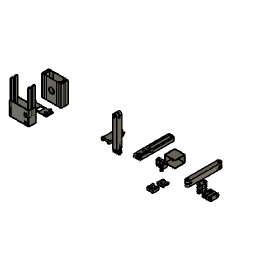
Table Lamp 3.0 v83 (Autodesk Fusion 360 design; units mm, degrees)
Autodesk Fusion 360 part; units mm, degrees
(part 1 of 3)
sketch "Schizzo1" plane through (0, 0, 0) normal (0, 0, 1) x (1, 0, 0)
  line L0 (-21, 0) -> (-5, 0)
  line L1 (-5, 0) -> (-5, 140)
  line L2 (-5, 140) -> (-21, 140)
  line L3 (-21, 140) -> (-21, 0)
  line L4 (-13, 140) -> (-13, 0)
  circle A0 centre (-13, 8) radius 8
  circle A1 centre (-13, 8) radius 4.1
  line L5 (-21, 70) -> (-5, 70)
  circle A2 centre (-13, 132) radius 8
  circle A3 centre (-13, 132) radius 4.1
  line L6 (26.1674, 0.6558) -> (42.1674, 0.6558)
  line L7 (42.1674, 0.6558) -> (42.1674, 33.6558)
  line L8 (42.1674, 33.6558) -> (26.1674, 33.6558)
  line L9 (26.1674, 33.6558) -> (26.1674, 0.6558)
  line L10 (34.1674, 0.6558) -> (34.1674, 33.6558)
  line L11 (26.1674, 17.1558) -> (42.1674, 17.1558)
  circle A4 centre (34.1674, 8.6558) radius 8
  arc A5 (42.1674, 11.5281) -> (34.1674, 17.1558) centre (34.1674, 8.6558) ccw
  circle A6 centre (34.1674, 25.6558) radius 8
  arc A7 (34.1674, 17.1558) -> (42.1674, 22.7835) centre (34.1674, 25.6558) ccw
  circle A8 centre (34.1674, 8.6558) radius 3.25
  line L12 (37.4174, 8.6519) -> (35.7958, 11.4684)
  line L13 (35.7958, 11.4684) -> (32.5458, 11.4724)
  line L14 (32.5458, 11.4724) -> (30.9174, 8.6597)
  line L15 (30.9174, 8.6597) -> (32.539, 5.8432)
  line L16 (32.539, 5.8432) -> (35.789, 5.8393)
  line L17 (35.789, 5.8393) -> (37.4174, 8.6519)
  line L18 (30.9174, 25.6519) -> (32.539, 28.4684)
  line L19 (32.539, 28.4684) -> (35.789, 28.4724)
  line L20 (35.789, 28.4724) -> (37.4174, 25.6597)
  line L21 (37.4174, 25.6597) -> (35.7958, 22.8432)
  line L22 (35.7958, 22.8432) -> (32.5458, 22.8393)
  line L23 (32.5458, 22.8393) -> (30.9174, 25.6519)
  circle A9 centre (34.1674, 8.6558) radius 1.6
  circle A10 centre (34.1674, 25.6558) radius 1.6
  circle A11 centre (-13, 8) radius 2
  circle A12 centre (-13, 132) radius 2
  line L24 (-130.5, 0) -> (-102.5, 0)
  line L25 (-102.5, 0) -> (-102.5, 16)
  line L26 (-102.5, 16) -> (-130.5, 16)
  line L27 (-130.5, 16) -> (-130.5, 0)
  line L28 (-116.5, 16) -> (-116.5, 0)
  line L29 (-130.5, 8) -> (-102.5, 8)
  line L30 (-130.5, 16) -> (-126.5, 16)
  line L31 (-126.5, 16) -> (-126.5, 0)
  line L32 (-126.5, 0) -> (-130.5, 0)
  line L33 (-130.5, 0) -> (-130.5, 16)
  line L34 (-106.5, 16) -> (-106.5, 0)
  line L35 (-115, 0) -> (-118, 0)
  line L36 (-118, 0) -> (-118, 16)
  line L37 (-118, 16) -> (-115, 16)
  line L38 (-115, 16) -> (-115, 0)
  line L39 (-115, 0) -> (-118, 16) construction
  line L40 (-118, 0) -> (-115, 16) construction
  line L41 (-114.5, 6) -> (-118.5, 6)
  line L42 (-118.5, 6) -> (-118.5, 10)
  line L43 (-118.5, 10) -> (-114.5, 10)
  line L44 (-114.5, 10) -> (-114.5, 6)
  line L45 (-114.5, 6) -> (-118.5, 10) construction
  line L46 (-118.5, 6) -> (-114.5, 10) construction
  line L47 (-114.5, 6) -> (-118.5, 6)
  line L48 (-118.5, 6) -> (-118.5, 10)
  line L49 (-118.5, 10) -> (-114.5, 10)
  line L50 (-114.5, 10) -> (-114.5, 6)
  line L51 (-114.5, 6) -> (-118.5, 10) construction
  line L52 (-118.5, 6) -> (-114.5, 10) construction
  circle A13 centre (-116.5, 8) radius 2.5
  line L53 (-135.9612, 39.7916) -> (-95.9612, 39.7916)
  line L54 (-95.9612, 39.7916) -> (-95.9612, 79.7916)
  line L55 (-95.9612, 79.7916) -> (-135.9612, 79.7916)
  line L56 (-135.9612, 79.7916) -> (-135.9612, 39.7916)
  circle A14 centre (-116.5, 8) radius 5
  circle A15 centre (-127.9112, 65.7416) radius 5.05
  line L57 (-132.9612, 79.7916) -> (-132.9612, 39.7916) construction
  line L58 (-135.9612, 79.7916) -> (-133.9612, 79.7916)
  line L59 (-133.9612, 79.7916) -> (-133.9612, 39.7916)
  line L60 (-133.9612, 39.7916) -> (-135.9612, 39.7916)
  line L61 (-135.9612, 39.7916) -> (-135.9612, 79.7916)
  line L62 (-135.9612, 79.7916) -> (-95.9612, 79.7916)
  line L63 (-95.9612, 79.7916) -> (-95.9612, 77.7916)
  line L64 (-95.9612, 77.7916) -> (-135.9612, 77.7916)
  line L65 (-135.9612, 77.7916) -> (-135.9612, 79.7916)
  line L66 (-135.9612, 70.7916) -> (-95.9612, 70.7916) construction
  line L67 (-95.9612, 65.7416) -> (-135.9612, 65.7416) construction
  line L68 (-78.8911, -24.4102) -> (-54.8911, -24.4102)
  line L69 (-54.8911, -24.4102) -> (-54.8911, -48.4102)
  line L70 (-54.8911, -48.4102) -> (-78.8911, -48.4102)
  line L71 (-78.8911, -48.4102) -> (-78.8911, -24.4102)
  line L72 (-78.8911, -38.4102) -> (-54.8911, -38.4102) construction
  line L73 (-75.8911, -24.4102) -> (-75.8911, -48.4102) construction
  circle A16 centre (-75.8911, -38.4102) radius 1.6
  line L74 (-66.8911, -24.4102) -> (-66.8911, -48.4102) construction
  circle A17 centre (-57.8911, -38.4102) radius 1.6
  circle A18 centre (-75.8911, -38.4102) radius 3 construction
  line L75 (-72.8911, -41.4102) -> (-78.8911, -41.4102)
  line L76 (-78.8911, -41.4102) -> (-78.8911, -35.4102)
  line L77 (-78.8911, -35.4102) -> (-72.8911, -35.4102)
  line L78 (-72.8911, -35.4102) -> (-72.8911, -41.4102)
  line L79 (-72.8911, -41.4102) -> (-78.8911, -35.4102) construction
  line L80 (-78.8911, -41.4102) -> (-72.8911, -35.4102) construction
  line L81 (-54.8911, -41.4102) -> (-54.8911, -35.4102)
  line L82 (-60.8911, -35.4102) -> (-60.8911, -41.4102)
  line L83 (-54.8911, -35.4102) -> (-60.8911, -35.4102)
  line L84 (-60.8911, -41.4102) -> (-54.8911, -41.4102)
  line L85 (-78.8911, -63.8199) -> (-54.8911, -63.8199)
  line L86 (-54.8911, -63.8199) -> (-54.8911, -87.8199)
  line L87 (-54.8911, -87.8199) -> (-78.8911, -87.8199)
  line L88 (-78.8911, -87.8199) -> (-78.8911, -63.8199)
  line L89 (-66.8911, -63.8199) -> (-66.8911, -87.8199) construction
  line L90 (-78.8911, -77.8199) -> (-54.8911, -77.8199) construction
  line L91 (-75.8911, -63.8199) -> (-75.8911, -87.8199) construction
  circle A19 centre (-75.8911, -77.8199) radius 1.4
  line L92 (-61.8911, -74.8199) -> (-71.8911, -74.8199)
  line L93 (-71.8911, -74.8199) -> (-71.8911, -63.8199)
  line L94 (-71.8911, -63.8199) -> (-61.8911, -63.8199)
  line L95 (-61.8911, -63.8199) -> (-61.8911, -74.8199)
  line L96 (-61.8911, -74.8199) -> (-71.8911, -63.8199) construction
  line L97 (-71.8911, -74.8199) -> (-61.8911, -63.8199) construction
  circle A20 centre (-57.8911, -77.8199) radius 1.4
  line L98 (-273.3139, -10.9044) -> (-253.3139, -10.9044)
  line L99 (-253.3139, -10.9044) -> (-253.3139, -30.9044)
  line L100 (-253.3139, -30.9044) -> (-273.3139, -30.9044)
  line L101 (-273.3139, -30.9044) -> (-273.3139, -10.9044)
  line L102 (-273.3139, -20.9044) -> (-253.3139, -20.9044)
  line L103 (-263.3139, -10.9044) -> (-263.3139, -30.9044)
  line L104 (-255.3139, -30.9044) -> (-271.3139, -30.9044)
  line L105 (-271.3139, -30.9044) -> (-271.3139, -10.9044)
  line L106 (-271.3139, -10.9044) -> (-255.3139, -10.9044)
  line L107 (-255.3139, -10.9044) -> (-255.3139, -30.9044)
  line L108 (-255.3139, -30.9044) -> (-271.3139, -10.9044) construction
  line L109 (-271.3139, -30.9044) -> (-255.3139, -10.9044) construction
  line L110 (-261.8139, -10.9044) -> (-264.8139, -10.9044)
  line L111 (-264.8139, -10.9044) -> (-264.8139, -30.9044)
  line L112 (-264.8139, -30.9044) -> (-261.8139, -30.9044)
  line L113 (-261.8139, -30.9044) -> (-261.8139, -10.9044)
  line L114 (-261.8139, -10.9044) -> (-264.8139, -30.9044) construction
  line L115 (-264.8139, -10.9044) -> (-261.8139, -30.9044) construction
  line L116 (-21, 12.1) -> (-5, 12.1)
  line L117 (-5, 12.1) -> (-5, 3.9)
  line L118 (-5, 3.9) -> (-21, 3.9)
  line L119 (-21, 3.9) -> (-21, 12.1)
  line L120 (-21, 12.1) -> (-5, 3.9) construction
  line L121 (-5, 12.1) -> (-21, 3.9) construction
  line L122 (-5, 136.1) -> (-21, 136.1)
  line L123 (-21, 136.1) -> (-21, 127.9)
  line L124 (-21, 127.9) -> (-5, 127.9)
  line L125 (-5, 127.9) -> (-5, 136.1)
  line L126 (60, 30) -> (88, 30)
  line L127 (88, 30) -> (88, -8)
  line L128 (88, -8) -> (60, -8)
  line L129 (60, -8) -> (60, 30)
  line L130 (74, 30) -> (74, -8)
  line L131 (60, 11) -> (88, 11)
  line L132 (60, 30) -> (64, 30)
  line L133 (64, 30) -> (64, -8)
  line L134 (64, -8) -> (60, -8)
  line L135 (60, -8) -> (60, 30)
  line L136 (88, 30) -> (84, 30)
  line L137 (84, -8) -> (88, -8)
  line L138 (88, -8) -> (88, 30)
  line L139 (84, 30) -> (84, -8)
  line L140 (75.5, -8) -> (72.5, -8)
  line L141 (72.5, -8) -> (72.5, 30)
  line L142 (72.5, 30) -> (75.5, 30)
  line L143 (75.5, 30) -> (75.5, -8)
  line L144 (75.5, -8) -> (72.5, 30) construction
  line L145 (72.5, -8) -> (75.5, 30) construction
  line L146 (88, 10) -> (60, 10)
  line L147 (60, 10) -> (60, 12)
  line L148 (60, 12) -> (88, 12)
  line L149 (88, 12) -> (88, 10)
  line L150 (88, 10) -> (60, 12) construction
  line L151 (60, 10) -> (88, 12) construction
  line L152 (-253.3139, -10.9044) -> (-257.3139, -10.9044) construction
  line L153 (-257.3139, -10.9044) -> (-257.3139, -15.9044) construction
  line L154 (-257.3139, -15.9044) -> (-253.3139, -15.9044) construction
  line L155 (-253.3139, -15.9044) -> (-253.3139, -10.9044) construction
  line L156 (-255.3139, -13.9044) -> (-259.3139, -13.9044)
  line L157 (-259.3139, -13.9044) -> (-259.3139, -17.9044)
  line L158 (-259.3139, -17.9044) -> (-255.3139, -17.9044)
  line L159 (-255.3139, -17.9044) -> (-255.3139, -13.9044)
  line L160 (-255.3139, -13.9044) -> (-259.3139, -17.9044) construction
  line L161 (-259.3139, -13.9044) -> (-255.3139, -17.9044) construction
  line L162 (-273.3139, -30.9044) -> (-267.8139, -30.9044) construction
  line L163 (-267.8139, -30.9044) -> (-267.8139, -26.9044) construction
  line L164 (-267.8139, -26.9044) -> (-273.3139, -26.9044) construction
  line L165 (-273.3139, -26.9044) -> (-273.3139, -30.9044) construction
  line L166 (-265.8139, -24.9044) -> (-269.8139, -24.9044)
  line L167 (-269.8139, -24.9044) -> (-269.8139, -28.9044)
  line L168 (-269.8139, -28.9044) -> (-265.8139, -28.9044)
  line L169 (-265.8139, -28.9044) -> (-265.8139, -24.9044)
  line L170 (-265.8139, -24.9044) -> (-269.8139, -28.9044) construction
  line L171 (-269.8139, -24.9044) -> (-265.8139, -28.9044) construction
  line L172 (-339.0462, -2) -> (-310.0462, -2)
  line L173 (-310.0462, -2) -> (-310.0462, 44.5)
  line L174 (-339.0462, 44.5) -> (-339.0462, -2)
  line L175 (-324.5462, 44.5) -> (-324.5462, -2)
  line L176 (-339.0462, 21.25) -> (-310.0462, 21.25)
  line L177 (-308.0462, 44.5) -> (-308.0462, 39.5)
  line L178 (-308.0462, 39.5) -> (-341.0462, 39.5)
  line L179 (-341.0462, 39.5) -> (-341.0462, 44.5)
  line L180 (-324.5462, 44.5) -> (-324.5462, 39.5)
  line L181 (-324.5462, 49.5) -> (-324.5462, 44.5) construction
  line L182 (-324.5462, 49.5) -> (-324.5462, 44.5) construction
  line L183 (-339.0462, -2) -> (-335.0462, -2)
  line L184 (-335.0462, -2) -> (-335.0462, -8)
  line L185 (-335.0462, -8) -> (-339.0462, -8)
  line L186 (-339.0462, -8) -> (-339.0462, -2)
  line L187 (-310.0462, -8) -> (-310.0462, -2)
  line L188 (-314.0462, -2) -> (-314.0462, -8)
  line L189 (-314.0462, -8) -> (-310.0462, -8)
  line L190 (-310.0462, -2) -> (-314.0462, -2)
  line L191 (-212.9415, -6.7942) -> (-192.9415, -6.7942)
  line L192 (-192.9415, -6.7942) -> (-192.9415, 133.2058)
  line L193 (-192.9415, 133.2058) -> (-212.9415, 133.2058)
  line L194 (-212.9415, 133.2058) -> (-212.9415, -6.7942)
  line L195 (-211.9415, 132.2058) -> (-193.9415, 132.2058)
  line L196 (-193.9415, 132.2058) -> (-193.9415, 40.2058)
  line L197 (-193.9415, 40.2058) -> (-211.9415, 40.2058)
  line L198 (-211.9415, 40.2058) -> (-211.9415, 132.2058)
  line L199 (-211.9415, 52.7058) -> (-193.9415, 52.7058)
  line L200 (-202.9415, -6.7942) -> (-202.9415, 133.2058) construction
  circle A21 centre (-202.9415, 26.7058) radius 5
  circle A22 centre (-202.9415, 26.7058) radius 3.25
  line L201 (-207.9415, 39.2058) -> (-197.9415, 39.2058)
  line L202 (-197.9415, 39.2058) -> (-197.9415, 14.2058)
  line L203 (-197.9415, 14.2058) -> (-207.9415, 14.2058)
  line L204 (-207.9415, 14.2058) -> (-207.9415, 39.2058)
  line L205 (-207.9415, 39.2058) -> (-197.9415, 14.2058) construction
  line L206 (-197.9415, 39.2058) -> (-207.9415, 14.2058) construction
  line L207 (-197.9415, 32.2058) -> (-200.9415, 32.2058)
  line L208 (-200.9415, 32.2058) -> (-200.9415, 39.2058)
  line L209 (-200.9415, 39.2058) -> (-197.9415, 39.2058)
  line L210 (-197.9415, 39.2058) -> (-197.9415, 32.2058)
  line L211 (-202.9415, 26.7058) -> (-192.9415, 26.7058) construction
  line L212 (-197.9415, 21.2058) -> (-200.9415, 21.2058)
  line L213 (-200.9415, 21.2058) -> (-200.9415, 14.2058)
  line L214 (-197.9415, 14.2058) -> (-197.9415, 21.2058)
  line L215 (-200.9415, 14.2058) -> (-197.9415, 14.2058)
  line L216 (-207.9415, 21.2058) -> (-204.9415, 21.2058)
  line L217 (-204.9415, 21.2058) -> (-204.9415, 14.2058)
  line L218 (-207.9415, 14.2058) -> (-207.9415, 21.2058)
  line L219 (-204.9415, 14.2058) -> (-207.9415, 14.2058)
  line L220 (-207.9415, 32.2058) -> (-204.9415, 32.2058)
  line L221 (-204.9415, 39.2058) -> (-207.9415, 39.2058)
  line L222 (-207.9415, 39.2058) -> (-207.9415, 32.2058)
  line L223 (-204.9415, 32.2058) -> (-204.9415, 39.2058)
  line L224 (-605.2788, 49.6443) -> (-528.2788, 49.6443)
  line L225 (-528.2788, 49.6443) -> (-528.2788, 21.6443)
  line L226 (-528.2788, 21.6443) -> (-605.2788, 21.6443)
  line L227 (-605.2788, 21.6443) -> (-605.2788, 49.6443)
  line L228 (-605.2788, 35.6443) -> (-528.2788, 35.6443)
  line L229 (-566.7788, 49.6443) -> (-566.7788, 21.6443)
  circle A23 centre (-583.2788, 35.6443) radius 13.5
  circle A24 centre (-550.2788, 35.6443) radius 13.5
  line L230 (-596.7788, 49.6443) -> (-596.7788, 21.6443)
  line L231 (-596.7788, 49.6443) -> (-596.7788, 21.6443)
  line L232 (-536.7788, 49.6443) -> (-536.7788, 21.6443)
  line L233 (-605.2788, 22.6443) -> (-528.2788, 22.6443)
  line L234 (-605.2788, 48.6443) -> (-528.2788, 48.6443)
  line L235 (-599.3788, 28.7443) -> (-595.2788, 28.7443)
  line L236 (-595.2788, 28.7443) -> (-595.2788, 22.5443)
  line L237 (-595.2788, 22.5443) -> (-599.3788, 22.5443)
  line L238 (-599.3788, 22.5443) -> (-599.3788, 28.7443)
  line L239 (-534.1788, 28.7443) -> (-538.2788, 28.7443)
  line L240 (-538.2788, 28.7443) -> (-538.2788, 22.5443)
  line L241 (-534.1788, 22.5443) -> (-534.1788, 28.7443)
  line L242 (-538.2788, 22.5443) -> (-534.1788, 22.5443)
  line L243 (-595.2788, 48.7443) -> (-599.3788, 48.7443)
  line L244 (-599.3788, 48.7443) -> (-599.3788, 42.5443)
  line L245 (-599.3788, 42.5443) -> (-595.2788, 42.5443)
  line L246 (-595.2788, 42.5443) -> (-595.2788, 48.7443)
  line L247 (-538.2788, 48.7443) -> (-534.1788, 48.7443)
  line L248 (-534.1788, 48.7443) -> (-534.1788, 42.5443)
  line L249 (-538.2788, 42.5443) -> (-538.2788, 48.7443)
  line L250 (-534.1788, 42.5443) -> (-538.2788, 42.5443)
  line L251 (-559.2788, 29.1443) -> (-574.2788, 29.1443)
  line L252 (-574.2788, 29.1443) -> (-574.2788, 42.1443)
  line L253 (-574.2788, 42.1443) -> (-559.2788, 42.1443)
  line L254 (-559.2788, 42.1443) -> (-559.2788, 29.1443)
  line L255 (-559.2788, 29.1443) -> (-574.2788, 42.1443) construction
  line L256 (-574.2788, 29.1443) -> (-559.2788, 42.1443) construction
  line L257 (-603.5788, 32.7443) -> (-599.3788, 32.7443)
  line L258 (-599.3788, 32.7443) -> (-599.3788, 22.5443)
  line L259 (-599.3788, 22.5443) -> (-603.5788, 22.5443)
  line L260 (-603.5788, 22.5443) -> (-603.5788, 32.7443)
  line L261 (-529.9788, 22.5443) -> (-529.9788, 32.7443)
  line L262 (-534.1788, 32.7443) -> (-534.1788, 22.5443)
  line L263 (-529.9788, 32.7443) -> (-534.1788, 32.7443)
  line L264 (-534.1788, 22.5443) -> (-529.9788, 22.5443)
  line L265 (-603.5788, 38.5443) -> (-599.3788, 38.5443)
  line L266 (-603.5788, 48.7443) -> (-603.5788, 38.5443)
  line L267 (-599.3788, 38.5443) -> (-599.3788, 48.7443)
  line L268 (-599.3788, 48.7443) -> (-603.5788, 48.7443)
  line L269 (-529.9788, 38.5443) -> (-534.1788, 38.5443)
  line L270 (-534.1788, 38.5443) -> (-534.1788, 48.7443)
  line L271 (-529.9788, 48.7443) -> (-529.9788, 38.5443)
  line L272 (-534.1788, 48.7443) -> (-529.9788, 48.7443)
  line L273 (-339.0462, 39.5) -> (-287, 39.5) construction
  line L274 (-312.1462, 44.5) -> (-318.8462, 44.5)
  line L275 (-318.8462, 44.5) -> (-318.8462, 54)
  line L276 (-318.8462, 54) -> (-312.1462, 54)
  line L277 (-312.1462, 54) -> (-312.1462, 44.5)
  line L278 (-308.0462, 44.5) -> (-341.0462, 44.5)
  line L279 (-336.9462, 54) -> (-336.9462, 44.5)
  line L280 (-330.2462, 44.5) -> (-330.2462, 54)
  line L281 (-336.9462, 44.5) -> (-330.2462, 44.5)
  line L282 (-330.2462, 54) -> (-336.9462, 54)
  line L283 (-308.0462, 44.5) -> (-314.0462, 44.5)
  line L284 (-314.0462, 44.5) -> (-314.0462, 54)
  line L285 (-314.0462, 54) -> (-308.0462, 54)
  line L286 (-308.0462, 54) -> (-308.0462, 44.5)
  line L287 (-335.0462, 54) -> (-341.0462, 54)
  line L288 (-335.0462, 44.5) -> (-335.0462, 54)
  line L289 (-341.0462, 54) -> (-341.0462, 44.5)
  line L290 (-341.0462, 44.5) -> (-335.0462, 44.5)
  line L291 (-605.2788, -9.4892) -> (-528.2788, -9.4892)
  line L292 (-528.2788, -9.4892) -> (-528.2788, -37.4892)
  line L293 (-528.2788, -37.4892) -> (-605.2788, -37.4892)
  line L294 (-605.2788, -37.4892) -> (-605.2788, -9.4892)
  line L295 (-566.7788, -9.4892) -> (-566.7788, -37.4892) construction
  line L296 (-605.2788, -23.4892) -> (-528.2788, -23.4892) construction
  line L297 (-559.2788, -13.4892) -> (-574.2788, -13.4892)
  line L298 (-574.2788, -13.4892) -> (-574.2788, -33.4892)
  line L299 (-574.2788, -33.4892) -> (-559.2788, -33.4892)
  line L300 (-559.2788, -33.4892) -> (-559.2788, -13.4892)
  line L301 (-559.2788, -13.4892) -> (-574.2788, -33.4892) construction
  line L302 (-574.2788, -13.4892) -> (-559.2788, -33.4892) construction
  line L303 (-605.2788, 48.6443) -> (-605.2788, -9.4892) construction
  line L304 (-599.2788, -16.4892) -> (-595.2788, -16.4892)
  line L305 (-595.2788, -16.4892) -> (-595.2788, -10.4892)
  line L306 (-595.2788, -10.4892) -> (-599.2788, -10.4892)
  line L307 (-599.2788, -10.4892) -> (-599.2788, -16.4892)
  line L308 (-603.4788, -10.4892) -> (-599.2788, -10.4892)
  line L309 (-599.2788, -10.4892) -> (-599.2788, -20.6892)
  line L310 (-599.2788, -20.6892) -> (-603.4788, -20.6892)
  line L311 (-603.4788, -20.6892) -> (-603.4788, -10.4892)
  line L312 (-534.2788, -20.6892) -> (-530.0788, -20.6892)
  line L313 (-534.2788, -10.4892) -> (-534.2788, -20.6892)
  line L314 (-530.0788, -20.6892) -> (-530.0788, -10.4892)
  line L315 (-530.0788, -10.4892) -> (-534.2788, -10.4892)
  line L316 (-538.2788, -10.4892) -> (-534.2788, -10.4892)
  line L317 (-538.2788, -16.4892) -> (-538.2788, -10.4892)
  line L318 (-534.2788, -16.4892) -> (-538.2788, -16.4892)
  line L319 (-599.2788, -26.2892) -> (-603.4788, -26.2892)
  line L320 (-603.4788, -26.2892) -> (-603.4788, -36.4892)
  line L321 (-603.4788, -36.4892) -> (-599.2788, -36.4892)
  line L322 (-595.2788, -36.4892) -> (-599.2788, -36.4892)
  line L323 (-595.2788, -30.4892) -> (-595.2788, -36.4892)
  line L324 (-599.2788, -30.4892) -> (-595.2788, -30.4892)
  line L325 (-599.2788, -36.4892) -> (-599.2788, -26.2892)
  line L326 (-534.2788, -30.4892) -> (-538.2788, -30.4892)
  line L327 (-538.2788, -30.4892) -> (-538.2788, -36.4892)
  line L328 (-534.2788, -36.4892) -> (-534.2788, -26.2892)
  line L329 (-538.2788, -36.4892) -> (-534.2788, -36.4892)
  line L330 (-530.0788, -36.4892) -> (-534.2788, -36.4892)
  line L331 (-530.0788, -26.2892) -> (-530.0788, -36.4892)
  line L332 (-534.2788, -26.2892) -> (-530.0788, -26.2892)
  line L333 (-589.2788, -25.4892) -> (-597.2788, -25.4892)
  line L334 (-597.2788, -25.4892) -> (-597.2788, -21.4892)
  line L335 (-597.2788, -21.4892) -> (-589.2788, -21.4892)
  line L336 (-589.2788, -21.4892) -> (-589.2788, -25.4892)
  line L337 (-589.2788, -25.4892) -> (-597.2788, -21.4892) construction
  line L338 (-597.2788, -25.4892) -> (-589.2788, -21.4892) construction
  line L339 (-536.2788, -25.4892) -> (-536.2788, -21.4892)
  line L340 (-536.2788, -21.4892) -> (-544.2788, -21.4892)
  line L341 (-544.2788, -25.4892) -> (-536.2788, -25.4892)
  line L342 (-544.2788, -21.4892) -> (-544.2788, -25.4892)
  line L343 (-528.2788, -78.2441) -> (-605.2788, -78.2441)
  line L344 (-605.2788, -78.2441) -> (-605.2788, -106.2441)
  line L345 (-605.2788, -106.2441) -> (-528.2788, -106.2441)
  line L346 (-528.2788, -106.2441) -> (-528.2788, -78.2441)
  line L347 (-603.2788, -79.2441) -> (-599.2788, -79.2441)
  line L348 (-599.2788, -79.2441) -> (-599.2788, -89.2441)
  line L349 (-599.2788, -89.2441) -> (-603.2788, -89.2441)
  line L350 (-603.2788, -89.2441) -> (-603.2788, -79.2441)
  line L351 (-566.7788, -78.2441) -> (-566.7788, -106.2441) construction
  line L352 (-528.2788, -92.2441) -> (-605.2788, -92.2441) construction
  line L353 (-603.2788, -104.2441) -> (-530.2788, -104.2441)
  line L354 (-530.2788, -104.2441) -> (-530.2788, -80.2441)
  line L355 (-530.2788, -80.2441) -> (-603.2788, -80.2441)
  line L356 (-603.2788, -80.2441) -> (-603.2788, -104.2441)
  line L357 (-530.2788, -89.2441) -> (-530.2788, -79.2441)
  line L358 (-534.2788, -79.2441) -> (-534.2788, -89.2441)
  line L359 (-530.2788, -79.2441) -> (-534.2788, -79.2441)
  line L360 (-534.2788, -89.2441) -> (-530.2788, -89.2441)
  line L361 (-603.2788, -95.2441) -> (-603.2788, -105.2441)
  line L362 (-603.2788, -105.2441) -> (-599.2788, -105.2441)
  line L363 (-599.2788, -105.2441) -> (-599.2788, -95.2441)
  line L364 (-599.2788, -95.2441) -> (-603.2788, -95.2441)
  line L365 (-534.2788, -95.2441) -> (-530.2788, -95.2441)
  line L366 (-530.2788, -105.2441) -> (-534.2788, -105.2441)
  line L367 (-534.2788, -105.2441) -> (-534.2788, -95.2441)
  line L368 (-530.2788, -95.2441) -> (-530.2788, -105.2441)
  line L369 (-542.2788, -78.2441) -> (-542.2788, -106.2441) construction
  line L370 (-542.2788, -94.2441) -> (-528.2788, -94.2441) construction
  circle A25 centre (-533.2788, -94.2441) radius 2.95
  circle A26 centre (-551.2788, -94.2441) radius 2.95
  line L371 (-551.2788, -94.2441) -> (-542.2788, -94.2441) construction
  line L372 (-330.2462, 44.5) -> (-318.8462, 44.5)
  line L373 (-318.8462, 44.5) -> (-318.8462, 38.5)
  line L374 (-318.8462, 38.5) -> (-330.2462, 38.5)
  line L375 (-330.2462, 38.5) -> (-330.2462, 44.5)
  line L376 (-324.5462, 44.5) -> (-324.5462, 38.5) construction
  point P0 (34.1674, 8.6558)
  point P1 (-116.5, 8)
  point P2 (-116.5, 8)
  point P3 (-116.5, 8)
  point P4 (-75.8911, -38.4102)
  point P5 (-54.8911, -38.4102)
  point P6 (-66.8911, -69.3199)
  point P7 (-263.3139, -20.9044)
  point P8 (-263.3139, -20.9044)
  point P9 (-13, 8)
  point P10 (74, 11)
  point P11 (74, 11)
  point P12 (-257.3139, -15.9044)
  point P13 (-267.8139, -26.9044)
  point P14 (-202.9415, 26.7058)
  point P15 (-566.7788, 35.6443)
  point P16 (-566.7788, -23.4892)
  point P17 (-593.2788, -23.4892)
  dimension "d2" = 140
  dimension "d3" = 16
  dimension "d4" = 8.2
  dimension "d16" = 16
  dimension "d17" = 33
  dimension "d19" = 6.5
  dimension "d26" = 3.2
  dimension "d75" = 4
  dimension "d139" = 28
  dimension "d140" = 16
  dimension "d141" = 4
  dimension "d142" = 3
  dimension "d149" = 4
  dimension "d150" = 4
  dimension "d177" = 4
  dimension "d180" = 5
  dimension "d182" = 40
  dimension "d183" = 40
  dimension "d184" = 10
  dimension "d186" = 10.1
  dimension "d191" = 3
  dimension "d192" = 2
  dimension "d195" = 2
  dimension "d198" = 9
  dimension "d257" = 24
  dimension "d258" = 24
  dimension "d261" = 3.2
  dimension "d262" = 10
  dimension "d264" = 9
  dimension "d265" = 6
  dimension "d279" = 24
  dimension "d280" = 24
  dimension "d281" = 10
  dimension "d282" = 9
  dimension "d283" = 2.8
  dimension "d284" = 10
  dimension "d285" = 11
  dimension "d305" = 20
  dimension "d306" = 20
  dimension "d307" = 16
  dimension "d313" = 3
  dimension "d360" = 28
  dimension "d361" = 38
  dimension "d362" = 3
  dimension "d363" = 4
  dimension "d364" = 2
  dimension "d388" = 4
  dimension "d389" = 5
  dimension "d390" = 4
  dimension "d391" = 4
  dimension "d394" = 5.5
  dimension "d395" = 4
  dimension "d396" = 4
  dimension "d397" = 4
  dimension "d420" = 29
  dimension "d422" = 33
  dimension "d423" = 5
  dimension "d442" = 4
  dimension "d443" = 6
  dimension "d459" = 20
  dimension "d460" = 140
  dimension "d474" = 1
  dimension "d475" = 1
  dimension "d476" = 1
  dimension "d477" = 92
  dimension "d478" = 12.5
  dimension "d485" = 10
  dimension "d486" = 6.5
  dimension "d487" = 13.5
  dimension "d488" = 25
  dimension "d496" = 3
  dimension "d497" = 7
  dimension "d527" = 77
  dimension "d528" = 28
  dimension "d529" = 27
  dimension "d530" = 33
  dimension "d531" = 60
  dimension "d532" = 1
  dimension "d535" = 4.1
  dimension "d536" = 6.2
  dimension "d537" = 0.9
  dimension "d538" = 5.9
  dimension "d539" = 15
  dimension "d540" = 13
  dimension "d550" = 4.2
  dimension "d551" = 10.2
  dimension "d553" = 5.7
  dimension "d554" = 6.7
  dimension "d555" = 24.8
  dimension "d556" = 11.4
  dimension "d557" = 6
  dimension "d558" = 9.5
  dimension "d559" = 9.5
  dimension "d566" = 77
  dimension "d567" = 28
  dimension "d568" = 15
  dimension "d569" = 20
  dimension "d570" = 4
  dimension "d571" = 6
  dimension "d572" = 1
  dimension "d573" = 6
  dimension "d574" = 4.2
  dimension "d575" = 10.2
  dimension "d580" = 8
  dimension "d581" = 4
  dimension "d582" = 8
  dimension "d586" = 21
  dimension "d587" = 77
  dimension "d588" = 28
  dimension "d589" = 4
  dimension "d590" = 10
  dimension "d591" = 6
  dimension "d592" = 1
  dimension "d593" = -2
  dimension "d610" = 14
  dimension "d611" = 12
  dimension "d612" = 5.9
  dimension "d613" = 9
  dimension "d627" = 11.4
  dimension "d628" = 6
  constraint horizontal L0
  constraint vertical L1
  constraint horizontal L2
  constraint vertical L3
  constraint midpoint L2 L4.start
  constraint midpoint L0 L4.end
  constraint coincident L4 P9
  constraint tangent L1 A0
  constraint tangent L0 A0
  constraint concentric A0 A1
  constraint midpoint L3 L5.start
  constraint midpoint L1 L5.end
  constraint symmetric A0 L5 A2
  constraint symmetric A1 L5 A3
  constraint horizontal L6
  constraint vertical L7
  constraint horizontal L8
  constraint vertical L9
  constraint midpoint L6 L10.start
  constraint midpoint L8 L10.end
  constraint midpoint L9 L11.start
  constraint midpoint L7 L11.end
  constraint coincident L10 P0
  constraint tangent L7 A4
  constraint tangent L6 A4
  constraint midpoint L11 A5.end
  constraint coincident P0 A4.centre
  constraint coincident L7 A5.start
  constraint symmetric L11 A4 A6
  constraint symmetric L11 A5.start A7.end
  constraint symmetric L11 A5.end A7.start
  constraint symmetric L11 A5 A7
  constraint concentric A5 A8
  constraint coincident A8 L12.start
  constraint symmetric L11 L12.start L20.end
  constraint symmetric L11 L12.end L21.end
  constraint symmetric L11 L13.end L22.end
  constraint symmetric L11 L14.end L18.start
  constraint symmetric L11 L15.end L18.end
  constraint symmetric L11 L16.end L19.end
  constraint symmetric L11 A9 A10
  constraint concentric A0 A11
  constraint symmetric L5 A11 A12
  constraint horizontal L24
  constraint vertical L25
  constraint horizontal L26
  constraint vertical L27
  constraint midpoint L26 L28.start
  constraint midpoint L24 L28.end
  constraint midpoint L27 L29.start
  constraint midpoint L25 L29.end
  constraint horizontal L30
  constraint vertical L31
  constraint horizontal L32
  constraint vertical L33
  constraint collinear L26 L30
  constraint collinear L24 L32
  constraint symmetric L28 L30.end L34.start
  constraint symmetric L28 L31.end L34.end
  constraint horizontal L35
  constraint perpendicular L35 L36
  constraint parallel L35 L37
  constraint parallel L36 L38
  constraint coincident L39 P3
  constraint coincident L40 P3
  constraint midpoint L29 P3
  constraint collinear L26 L37
  constraint collinear L27 L33
  constraint horizontal L41
  constraint perpendicular L41 L42
  constraint parallel L41 L43
  constraint parallel L42 L44
  constraint coincident L45 P3
  constraint coincident L46 P3
  constraint coincident P3 P2
  constraint horizontal L47
  constraint perpendicular L47 L48
  constraint parallel L47 L49
  constraint parallel L48 L50
  constraint coincident L51 P3
  constraint coincident L52 P3
  constraint collinear L43 L49
  constraint horizontal L53
  constraint vertical L54
  constraint horizontal L55
  constraint vertical L56
  constraint concentric A13 A14
  constraint coincident L55 L57.start
  constraint coincident L53 L57.end
  constraint perpendicular L53 L57
  constraint tangent A15 L57
  constraint horizontal L58
  constraint vertical L59
  constraint horizontal L60
  constraint vertical L61
  constraint coincident L53.start L56.end
  constraint horizontal L62
  constraint vertical L63
  constraint horizontal L64
  constraint vertical L65
  constraint coincident L54.end L55.start
  constraint coincident L61 L66.start
  constraint coincident L54 L66.end
  constraint perpendicular L54 L66
  constraint tangent A15 L66
  constraint coincident L54 L67.start
  constraint coincident L61 L67.end
  constraint perpendicular L61 L67
  constraint coincident A15.centre L67
  constraint horizontal L68
  constraint vertical L69
  constraint horizontal L70
  constraint vertical L71
  constraint coincident L71 L72.start
  constraint coincident L69 P5
  constraint perpendicular L69 L72
  constraint coincident L68 L73.start
  constraint coincident L70 L73.end
  constraint perpendicular L70 L73
  constraint coincident L73 P4
  constraint coincident L72 P4
  constraint midpoint L68 L74.start
  constraint midpoint L70 L74.end
  constraint symmetric A16 L74 A17
  constraint concentric A16 A18
  constraint horizontal L75
  constraint perpendicular L75 L76
  constraint parallel L75 L77
  constraint parallel L76 L78
  constraint coincident L79 P4
  constraint coincident L80 P4
  constraint coincident P4 A16.centre
  constraint collinear L71 L76
  constraint tangent A18 L75
  constraint symmetric L72.start L74 P5
  constraint symmetric L74 L75.start L82.end
  constraint symmetric L74 L75.end L81.start
  constraint symmetric L74 L76.end L81.end
  constraint symmetric L74 L77.end L82.start
  constraint horizontal L85
  constraint vertical L86
  constraint horizontal L87
  constraint vertical L88
  constraint midpoint L85 L89.start
  constraint midpoint L87 L89.end
  constraint coincident L88 L90.start
  constraint coincident L86 L90.end
  constraint perpendicular L86 L90
  constraint coincident L85 L91.start
  constraint coincident L87 L91.end
  constraint perpendicular L87 L91
  constraint collinear L74 L89
  constraint coincident L91 A19.centre
  constraint coincident L90 A19.centre
  constraint horizontal L92
  constraint perpendicular L92 L93
  constraint parallel L92 L94
  constraint parallel L93 L95
  constraint coincident L96 P6
  constraint coincident L97 P6
  constraint coincident L89 P6
  constraint collinear L85 L94
  constraint symmetric L89 A19 A20
  constraint horizontal L98
  constraint vertical L99
  constraint horizontal L100
  constraint vertical L101
  constraint midpoint L101 L102.start
  constraint midpoint L99 L102.end
  constraint midpoint L98 L103.start
  constraint midpoint L100 L103.end
  constraint horizontal L104
  constraint perpendicular L104 L105
  constraint parallel L104 L106
  constraint parallel L105 L107
  constraint coincident L108 P8
  constraint coincident L109 P8
  constraint midpoint L103 P8
  constraint collinear L98 L106
  constraint horizontal L110
  constraint perpendicular L110 L111
  constraint parallel L110 L112
  constraint parallel L111 L113
  constraint coincident L114 P8
  constraint coincident L115 P8
  constraint coincident P8 P7
  constraint collinear L106 L110
  constraint horizontal L116
  constraint perpendicular L116 L117
  constraint parallel L116 L118
  constraint parallel L117 L119
  constraint coincident L120 P9
  constraint coincident L121 P9
  constraint coincident P9 A0.centre
  constraint symmetric L5 L116.start L123.end
  constraint symmetric L5 L116.end L124.end
  constraint symmetric L5 L117.end L122.start
  constraint symmetric L5 L118.end L122.end
  constraint tangent A1 L118
  constraint tangent A0 L117
  constraint horizontal L126
  constraint vertical L127
  constraint horizontal L128
  constraint vertical L129
  constraint midpoint L126 L130.start
  constraint midpoint L128 L130.end
  constraint midpoint L129 L131.start
  constraint midpoint L127 L131.end
  constraint horizontal L132
  constraint vertical L133
  constraint horizontal L134
  constraint vertical L135
  constraint symmetric L130 L126.start L126.end
  constraint symmetric L130 L132.end L136.end
  constraint symmetric L130 L133.end L137.start
  constraint symmetric L130 L128.end L127.end
  constraint coincident L126.start L135
  constraint collinear L128 L134
  constraint horizontal L140
  constraint perpendicular L140 L141
  constraint parallel L140 L142
  constraint parallel L141 L143
  constraint coincident L144 P11
  constraint coincident L145 P11
  constraint midpoint L130 P11
  constraint collinear L126 L142
  constraint horizontal L146
  constraint perpendicular L146 L147
  constraint parallel L146 L148
  constraint parallel L147 L149
  constraint coincident L150 P11
  constraint coincident L151 P11
  constraint coincident P11 P10
  constraint collinear L135 L147
  constraint horizontal L152
  constraint vertical L153
  constraint horizontal L154
  constraint vertical L155
  constraint horizontal L156
  constraint perpendicular L156 L157
  constraint parallel L156 L158
  constraint parallel L157 L159
  constraint coincident L160 P12
  constraint coincident L161 P12
  constraint coincident P12 L153.end
  constraint horizontal L162
  constraint vertical L163
  constraint horizontal L164
  constraint vertical L165
  constraint horizontal L166
  constraint perpendicular L166 L167
  constraint parallel L166 L168
  constraint parallel L167 L169
  constraint coincident L170 P13
  constraint coincident L171 P13
  constraint coincident P13 L163.end
  constraint horizontal L172
  constraint vertical L173
  constraint vertical L174
  constraint midpoint L172 L175.end
  constraint midpoint L174 L176.start
  constraint midpoint L173 L176.end
  constraint vertical L177
  constraint horizontal L178
  constraint vertical L179
  constraint midpoint L178 L180.end
  constraint coincident L175.start L180.start
  constraint coincident L181.start L182.start
  constraint horizontal L183
  constraint vertical L184
  constraint horizontal L185
  constraint vertical L186
  constraint symmetric L172.start L175 L172.end
  constraint symmetric L175 L183.end L188.start
  constraint symmetric L175 L184.end L188.end
  constraint symmetric L175 L185.end L187.start
  constraint horizontal L191
  constraint vertical L192
  constraint horizontal L193
  constraint vertical L194
  constraint horizontal L195
  constraint vertical L196
  constraint horizontal L197
  constraint vertical L198
  constraint coincident L198 L199.start
  constraint coincident L196 L199.end
  constraint perpendicular L196 L199
  constraint midpoint L191 L200.start
  constraint midpoint L193 L200.end
  constraint coincident L200 P14
  constraint concentric A21 A22
  constraint horizontal L201
  constraint perpendicular L201 L202
  constraint parallel L201 L203
  constraint parallel L202 L204
  constraint coincident L205 P14
  constraint coincident L206 P14
  constraint coincident P14 A21.centre
  constraint tangent A21 L202
  constraint horizontal L207
  constraint vertical L208
  constraint horizontal L209
  constraint vertical L210
  constraint coincident L192 L211.end
  constraint perpendicular L192 L211
  constraint symmetric L207.start L211 L212.start
  constraint symmetric L207.end L211 L212.end
  constraint symmetric L208.end L211 L213.end
  constraint symmetric L201.end L211 L202.end
  constraint symmetric L200 L207.start L220.start
  constraint symmetric L200 L207.end L220.end
  constraint symmetric L200 L208.end L221.start
  constraint symmetric L200 L201.end L201.start
  constraint symmetric L200 L212.start L216.start
  constraint symmetric L200 L212.end L216.end
  constraint symmetric L200 L213.end L217.end
  constraint symmetric L200 L202.end L203.end
  constraint coincident L201.end L202.start
  constraint horizontal L224
  constraint vertical L225
  constraint horizontal L226
  constraint vertical L227
  constraint midpoint L227 L228.start
  constraint midpoint L225 L228.end
  constraint midpoint L224 L229.start
  constraint midpoint L226 L229.end
  constraint coincident L228 A23.centre
  constraint symmetric L229 A23 A24
  constraint coincident L224 L230.start
  constraint coincident L226 L230.end
  constraint perpendicular L226 L230
  constraint symmetric L231.start L230 L230.start
  constraint symmetric L231.end L230 L230.end
  constraint tangent A23 L230
  constraint symmetric L229 L230.start L232.start
  constraint symmetric L229 L230.end L232.end
  constraint coincident L227 L233.start
  constraint coincident L225 L233.end
  constraint perpendicular L225 L233
  constraint symmetric L228 L233.start L234.start
  constraint symmetric L228 L233.end L234.end
  constraint horizontal L235
  constraint vertical L236
  constraint horizontal L237
  constraint vertical L238
  constraint symmetric L229 L235.start L239.start
  constraint symmetric L229 L235.end L239.end
  constraint symmetric L229 L236.end L240.end
  constraint symmetric L229 L237.end L241.start
  constraint symmetric L228 L235.start L244.end
  constraint symmetric L228 L235.end L245.end
  constraint symmetric L228 L236.end L243.start
  constraint symmetric L228 L237.end L243.end
  constraint symmetric L228 L239.start L248.end
  constraint symmetric L228 L239.end L249.start
  constraint symmetric L228 L240.end L247.start
  constraint symmetric L228 L241.start L247.end
  constraint horizontal L251
  constraint perpendicular L251 L252
  constraint parallel L251 L253
  constraint parallel L252 L254
  constraint coincident L255 P15
  constraint coincident L256 P15
  constraint midpoint L229 P15
  constraint horizontal L257
  constraint vertical L258
  constraint horizontal L259
  constraint vertical L260
  constraint horizontal L237.end L238.start
  constraint collinear L238 L258
  constraint symmetric L229 L257.start L261.end
  constraint symmetric L229 L257.end L262.start
  constraint symmetric L229 L259.end L261.start
  constraint symmetric L228 L257.start L265.start
  constraint symmetric L228 L257.end L265.end
  constraint symmetric L228 L259.end L266.start
  constraint symmetric L228 L261.start L271.start
  constraint symmetric L228 L261.end L269.start
  constraint symmetric L228 L262.start L269.end
  constraint coincident L178 L273.start
  constraint coincident L174 L273.start
  constraint perpendicular L174 L273
  constraint horizontal L274
  constraint vertical L275
  constraint horizontal L276
  constraint vertical L277
  constraint perpendicular L179 L278
  constraint collinear L274 L278
  constraint symmetric L181 L274.start L279.end
  constraint symmetric L181 L274.end L280.start
  constraint symmetric L181 L275.end L280.end
  constraint symmetric L181 L276.end L279.start
  constraint horizontal L283
  constraint vertical L284
  constraint horizontal L285
  constraint vertical L286
  constraint coincident L177.start L278.start
  constraint symmetric L181 L177.start L179.end
  constraint symmetric L181 L283.end L288.start
  constraint symmetric L181 L284.end L287.start
  constraint symmetric L181 L285.end L287.end
  constraint horizontal L291
  constraint vertical L292
  constraint horizontal L293
  constraint vertical L294
  constraint midpoint L291 L295.start
  constraint midpoint L293 L295.end
  constraint midpoint L294 L296.start
  constraint midpoint L292 L296.end
  constraint horizontal L297
  constraint perpendicular L297 L298
  constraint parallel L297 L299
  constraint parallel L298 L300
  constraint coincident L301 P16
  constraint coincident L302 P16
  constraint midpoint L295 P16
  constraint perpendicular L293 L303
  constraint coincident L291.start L294.end
  constraint horizontal L304
  constraint vertical L305
  constraint horizontal L306
  constraint vertical L307
  constraint horizontal L308
  constraint vertical L309
  constraint horizontal L310
  constraint vertical L311
  constraint coincident L306.end L307.start
  constraint symmetric L295 L304.start L318.start
  constraint symmetric L295 L304.end L317.start
  constraint symmetric L295 L305.end L316.start
  constraint symmetric L295 L306.end L313.start
  constraint symmetric L295 L308.start L314.end
  constraint symmetric L295 L309.end L312.start
  constraint symmetric L295 L310.end L312.end
  constraint symmetric L296 L304.start L324.start
  constraint symmetric L296 L304.end L323.start
  constraint symmetric L296 L305.end L322.start
  constraint symmetric L296 L306.end L321.end
  constraint symmetric L296 L308.start L320.end
  constraint symmetric L296 L309.end L319.start
  constraint symmetric L296 L310.end L319.end
  constraint symmetric L296 L312.start L328.end
  constraint symmetric L296 L312.end L331.start
  constraint symmetric L296 L313.start L328.start
  constraint symmetric L296 L314.end L330.start
  constraint symmetric L296 L316.start L327.end
  constraint symmetric L296 L317.start L326.end
  constraint symmetric L296 L318.start L326.start
  constraint horizontal L333
  constraint perpendicular L333 L334
  constraint parallel L333 L335
  constraint parallel L334 L336
  constraint coincident L337 P17
  constraint coincident L338 P17
  constraint coincident L296 P17
  constraint symmetric L295 L333.start L341.start
  constraint symmetric L295 L333.end L339.start
  constraint symmetric L295 L334.end L339.end
  constraint symmetric L295 L335.end L340.end
  constraint horizontal L343
  constraint vertical L344
  constraint horizontal L345
  constraint vertical L346
  constraint collinear L292 L346
  constraint horizontal L347
  constraint vertical L348
  constraint horizontal L349
  constraint vertical L350
  constraint midpoint L343 L351.start
  constraint midpoint L345 L351.end
  constraint midpoint L346 L352.start
  constraint midpoint L344 L352.end
  constraint symmetric L347.start L351 L357.end
  constraint symmetric L347.end L351 L358.start
  constraint symmetric L348.end L351 L358.end
  constraint symmetric L349.end L351 L357.start
  constraint symmetric L347.start L352 L361.end
  constraint symmetric L347.end L352 L362.end
  constraint symmetric L348.end L352 L363.end
  constraint symmetric L349.end L352 L361.start
  constraint symmetric L352 L357.start L365.end
  constraint symmetric L352 L357.end L366.start
  constraint symmetric L352 L358.start L366.end
  constraint symmetric L352 L358.end L365.start
  constraint coincident L343 L369.start
  constraint coincident L345 L369.end
  constraint perpendicular L345 L369
  constraint coincident L369 L370.start
  constraint coincident L346 L370.end
  constraint perpendicular L346 L370
  constraint coincident L370 A25.centre
  constraint symmetric L369 A25 A26
  constraint coincident A26.centre L371.start
  constraint horizontal L372
  constraint vertical L373
  constraint horizontal L374
  constraint vertical L375
  constraint midpoint L372 L175.start
  constraint midpoint L374 L376.end
  measures "d2" distance of L0 L2
  measures "d3" diameter of A0
  measures "d4" diameter of A1
  measures "d16" distance of L6.start L6.end
  measures "d17" distance of L6.start L8.end
  measures "d19" diameter of A8
  measures "d26" diameter of A9
  measures "d75" diameter of A11
  measures "d139" distance of L24.start L24.end
  measures "d140" distance of L24.start L26.end
  measures "d141" distance of L31 L33
  measures "d142" distance of L36 L38
  measures "d149" distance of L42.end L43.end
  measures "d150" distance of L41.end L42.end
  measures "d177" distance of L42.end L43.end
  measures "d180" diameter of A13
  measures "d182" distance of L53.start L53.end
  measures "d183" distance of L53.start L55.end
  measures "d184" diameter of A14
  measures "d186" diameter of A15
  measures "d191" distance of L56 L57
  measures "d192" distance of L55.end L58.end
  measures "d195" distance of L62 L64
  measures "d198" distance of L55 L66
  measures "d257" distance of L68.start L68.end
  measures "d258" distance of L68.start L70.end
  measures "d261" diameter of A16
  measures "d262" distance of L70 L72
  measures "d264" distance of L73 L74
  measures "d265" diameter of A18
  measures "d279" distance of L85.start L85.end
  measures "d280" distance of L85.start L87.end
  measures "d281" distance of L87 L90
  measures "d282" distance of L89 L91
  measures "d283" diameter of A19
  measures "d284" distance of L93.end L94.end
  measures "d285" distance of L92.end L93.end
  measures "d305" distance of L98.start L98.end
  measures "d306" distance of L98.start L100.end
  measures "d307" distance of L105.end L106.end
  measures "d313" distance of L111 L113
  measures "d360" distance of L126.start L126.end
  measures "d361" distance of L126.end L127.end
  measures "d362" distance of L141.end L142.end
  measures "d363" distance of L129 L133
  measures "d364" distance of L146.end L147.end
  measures "d388" distance of L98.end L152.end
  measures "d389" distance of L98.end L154.end
  measures "d390" distance of L157.end L158.end
  measures "d391" distance of L156.end L157.end
  measures "d394" distance of L100.end L162.end
  measures "d395" distance of L100.end L164.end
  measures "d396" distance of L167.end L168.end
  measures "d397" distance of L166.end L167.end
  measures "d420" distance of L172.start L172.end
  measures "d422" distance of L179.end L177.start
  measures "d423" distance of L179.end L178.end
  measures "d442" distance of L172.start L183.end
  measures "d443" distance of L172.start L185.end
  measures "d459" distance of L191.start L191.end
  measures "d460" distance of L191.start L193.end
  measures "d474" distance of L193 L195
  measures "d475" distance of L194 L198
  measures "d476" distance of L192 L196
  measures "d477" distance of L195 L197
  measures "d478" distance of L197 L199
  measures "d485" diameter of A21
  measures "d486" diameter of A22
  measures "d487" distance of L197 P14
  measures "d488" distance of L201 L203
  measures "d496" distance of L207.start L207.end
  measures "d497" distance of L207.start L201.end
  measures "d527" distance of L224.start L224.end
  measures "d528" distance of L224.start L226.end
  measures "d529" diameter of A23
  measures "d530" distance of A23.centre A24.centre
  measures "d531" distance of L230 L232
  measures "d532" distance of L226 L233
  measures "d535" distance of L235.start L235.end
  measures "d536" distance of L235.start L237.end
  measures "d537" distance of L226 L237.end
  measures "d538" distance of L227 L237.end
  measures "d539" distance of L252.end L253.end
  measures "d540" distance of L251.end L252.end
  measures "d550" distance of L257.start L257.end
  measures "d551" distance of L257.start L259.end
  measures "d553" distance of L181 L275
  measures "d554" distance of L275 L277
  measures "d555" distance of L277 L279
  measures "d556" distance of L275 L280
  measures "d557" distance of L177.start L283.end
  measures "d558" distance of L177.start L285.end
  measures "d559" vertical distance of L179.end L279.start
  measures "d566" distance of L291.start L291.end
  measures "d567" distance of L291.start L293.end
  measures "d568" distance of L298.end L299.end
  measures "d569" distance of L297.end L298.end
  measures "d570" distance of L304.start L304.end
  measures "d571" distance of L304.start L306.end
  measures "d572" distance of L291 L306
  measures "d573" distance of L294 L307
  measures "d574" distance of L308.start L306.end
  measures "d575" distance of L308.start L310.end
  measures "d580" distance of L334.end L335.end
  measures "d581" distance of L333.end L334.end
  measures "d582" distance of L294 L334
  measures "d586" distance of L191 L203.end
  measures "d587" distance of L343.start L343.end
  measures "d588" distance of L343.start L345.end
  measures "d589" distance of L347.start L347.end
  measures "d590" distance of L347.start L349.end
  measures "d591" distance of L344 L348
  measures "d592" distance of L343 L347
  measures "d610" distance of L346 L369
  measures "d611" distance of L345 L370
  measures "d612" diameter of A25
  measures "d613" distance of L369 A25.centre
  measures "d627" distance of L280.start L274.end
  measures "d628" distance of L280.start L374.end
extrude "Estrusione1" add sketch "Schizzo1" along normal blind 20 contours L0 L3 A0 L118 | L0 L1 A0 L118 | L4 A0 L118 | L4 A0 L118 | L3 A0 L118 L119 | L4 A1 A11 | A0 A1 L116 L118 | L4 A1 A11 | A0 A1 L116 L118 | L1 A0 L117 L118 | L3 A0 L116 L119 | L4 A0 L116 | L4 A0 L116 | L1 A0 L116 L117 | L3 L4 A0 L5 L116 | L1 L4 A0 L5 L116 | L3 L4 L5 A2 L124 | L1 L4 L5 A2 L124 | L3 A2 L123 L124 | L4 A2 L124 | L4 A2 L124 | L1 A2 L124 L125 | L3 A2 L122 L123 | A2 A3 L122 L124 | L4 A3 A12 | L4 A3 A12 | A2 A3 L122 L124 | L1 A2 L122 L125 | L2 L3 A2 L122 | L4 A2 L122 | L4 A2 L122 | L1 L2 A2 L122 makes body 1